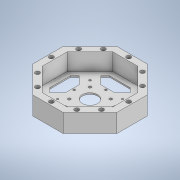
# Autodesk Inventor part: Base_Lid
Saved by Autodesk Inventor 2022 (Build 260153000, 153)
## iProperties
Created: 2022-03-24
Part Number: Base_Lid
Material: Generic
Document SubType Name: Modeling
Designer: Mlees
Density: 1 g/cm^3
Appearance: Default
Author: Mlees
Autodesk Inventor part; units mm, degrees
ref_plane "YZ Plane" through (0, 0, 0) normal (1, 0, 0) x (0, 1, 0)
ref_plane "XZ Plane" through (0, 0, 0) normal (0, 1, 0) x (-1, 0, 0)
ref_plane "XY Plane" through (0, 0, 0) normal (0, 0, 1) x (1, 0, 0)
sketch "Sketch1" plane through (0, 0, 0) normal (0, 1, 0) x (-1, 0, 0)
  line L0 (0, 0) -> (0, 22.75)
  line L1 (40, 62.75) -> (0, 22.75)
  line L2 (40, 62.75) -> (85.5, 62.75)
  line L3 (85.5, 62.75) -> (125.5, 22.75)
  line L4 (125.5, 22.75) -> (125.5, 0)
  line L5 (0, 0) -> (0, -22.75)
  line L6 (40, -62.75) -> (0, -22.75)
  line L7 (40, -62.75) -> (85.5, -62.75)
  line L8 (85.5, -62.75) -> (125.5, -22.75)
  line L9 (125.5, -22.75) -> (125.5, 0)
  dimension "d0" = 22.75
  dimension "d3" = 45.5
  dimension "d4" = 135
  constraints: 20 end point, 1 horizontal, 1 perpendicular, 1 vertical
  measures "d0" distance of L0.start L0.end
  measures "d3" distance of L1.start L2.end
  measures "d4" angle of L2 L3
extrude "Extrusion1" add sketch "Sketch1" along normal blind 2
sketch "Sketch2" plane through (0, 2, 0) normal (0, 1, 0) x (1, 0, 0)
  line L0 (-85.5, -62.75) -> (-40, -62.75) projected
  line L1 (-62.75, -62.75) -> (-62.75, 0)
  circle A0 centre (-62.75, 0) radius 11.5
  point P0 (0, 0)
  point P1 (-78.25, -15.5)
  point P2 (-47.25, -15.5)
  point P3 (-47.25, 15.5)
  point P4 (-78.25, 15.5)
  dimension "d7" = 23
  constraints: 2 end point, 1 centre point, 1 coincident, 1 midpoint, 1 vertical
  measures "d7" diameter of A0
extrude "Extrusion2" cut sketch "Sketch2" against normal blind 2
sketch "Sketch3" plane through (0, 2, 0) normal (0, 1, 0) x (1, 0, 0)
  circle A0 centre (-62.75, 0) radius 11.5 projected
  point P0 (0, 0)
  point P1 (-78.25, -15.5)
  point P2 (-47.25, -15.5)
  point P3 (-47.25, 15.5)
  point P4 (-78.25, 15.5)
hole "Hole1" at (-78.25, 2, 15.5) at (-47.25, 2, 15.5) at (-47.25, 2, -15.5) at (-78.25, 2, -15.5) direction (0, -1, 0) diameter 4 depth 2 tip angle 118
sketch "Sketch4" plane through (0, 2, 0) normal (0, 1, 0) x (1, 0, 0)
  line L0 (-125.5, -22.75) -> (-85.5, -62.75) projected
  line L1 (-85.5, -62.75) -> (-125.5, -22.75)
  line L2 (-125.5, 22.75) -> (-125.5, -22.75) projected
  line L3 (-125.5, -22.75) -> (-125.5, 22.75)
  line L4 (-85.5, 62.75) -> (-125.5, 22.75) projected
  line L5 (-125.5, 22.75) -> (-85.5, 62.75)
  line L6 (-40, 62.75) -> (-85.5, 62.75) projected
  line L7 (-85.5, 62.75) -> (-40, 62.75)
  line L8 (0, -22.75) -> (0, 22.75) projected
  line L9 (-40, 62.75) -> (0, 22.75)
  line L10 (0, 22.75) -> (0, -22.75)
  line L11 (-40, -62.75) -> (0, -22.75) projected
  line L12 (0, -22.75) -> (-40, -62.75)
  line L13 (-85.5, -62.75) -> (-40, -62.75) projected
  line L14 (-40, -62.75) -> (-85.5, -62.75)
  circle A0 centre (-62.75, 0) radius 11.5 projected
  point P0 (0, 0)
  point P1 (-62.75, -57.75)
  point P2 (-92.0542, -49.1247)
  point P3 (-110.5001, -30.6788)
  point P4 (-33.4458, -49.1247)
  point P5 (-14.9999, -30.6788)
  point P6 (-5, 0)
  point P7 (-120.5, 0)
  point P8 (-62.75, 57.75)
  point P9 (-92.0542, 49.1247)
  point P10 (-110.5001, 30.6788)
  point P11 (-33.4458, 49.1247)
  point P12 (-14.9999, 30.6788)
  constraints: 16 end point, 8 equal length
hole "Hole2" at (-62.75, 2, 57.75) at (-92.0542, 2, 49.1247) at (-110.5001, 2, 30.6788) at (-33.4458, 2, 49.1247) at (-14.9999, 2, 30.6788) at (-5, 2, 0) at (-120.5, 2, 0) at (-110.5001, 2, -30.6788) at (-92.0542, 2, -49.1247) at (-62.75, 2, -57.75) at (-33.4458, 2, -49.1247) at (-14.9999, 2, -30.6788) direction (0, -1, 0) diameter 4 depth 2 tip angle 118
sketch "Sketch5" plane through (0, 2, 0) normal (0, 1, 0) x (1, 0, 0)
  line L0 (-40, -62.75) -> (0, -22.75) projected
  line L1 (-85.5, -62.75) -> (-40, -62.75) projected
  line L2 (-40, -62.75) -> (-85.5, -62.75)
  line L3 (-125.5, 22.75) -> (-125.5, -22.75) projected
  line L4 (-85.5, -62.75) -> (-125.5, -22.75)
  line L5 (-125.5, -22.75) -> (-125.5, 22.75)
  line L6 (-85.5, 62.75) -> (-125.5, 22.75) projected
  line L7 (-125.5, 22.75) -> (-85.5, 62.75)
  line L8 (-40, 62.75) -> (-85.5, 62.75) projected
  line L9 (-85.5, 62.75) -> (-40, 62.75)
  line L10 (0, -22.75) -> (0, 22.75) projected
  line L11 (-40, 62.75) -> (0, 22.75)
  line L12 (0, 22.75) -> (0, -22.75)
  line L13 (0, -22.75) -> (-40, -62.75)
  line L14 (-81.3579, -52.75) -> (-44.1421, -52.75)
  line L15 (-10, -18.6079) -> (-10, 18.6079)
  line L16 (-44.1421, 52.75) -> (-81.3579, 52.75)
  line L17 (-115.5, 18.6079) -> (-115.5, -18.6079)
  line L18 (-49.1421, -18.6079) -> (-76.3579, -18.6079)
  line L19 (-81.3579, -13.6079) -> (-81.3579, 13.6079)
  line L20 (-76.3579, 18.6079) -> (-49.1421, 18.6079)
  line L21 (-44.1421, 13.6079) -> (-44.1421, -13.6079)
  line L22 (-44.1421, -13.6079) -> (-24.5711, -33.1789)
  line L23 (-49.1421, -18.6079) -> (-29.5711, -38.1789)
  line L24 (-76.3579, -18.6079) -> (-95.9289, -38.1789)
  line L25 (-81.3579, -13.6079) -> (-100.9289, -33.1789)
  line L26 (-81.3579, 13.6079) -> (-100.9289, 33.1789)
  line L27 (-76.3579, 18.6079) -> (-95.9289, 38.1789)
  line L28 (-49.1421, 18.6079) -> (-29.5711, 38.1789)
  line L29 (-44.1421, 13.6079) -> (-24.5711, 33.1789)
  line L30 (-115.5, -18.6079) -> (-100.9289, -33.1789)
  line L31 (-95.9289, -38.1789) -> (-81.3579, -52.75)
  line L32 (-44.1421, -52.75) -> (-29.5711, -38.1789)
  line L33 (-24.5711, -33.1789) -> (-10, -18.6079)
  line L34 (-10, 18.6079) -> (-24.5711, 33.1789)
  line L35 (-29.5711, 38.1789) -> (-44.1421, 52.75)
  line L36 (-91.6863, -38.1789) -> (-75.1152, -21.6079)
  line L37 (-75.1152, -21.6079) -> (-50.3848, -21.6079)
  line L38 (-50.3848, -21.6079) -> (-33.8137, -38.1789)
  line L39 (-33.8137, -38.1789) -> (-45.3848, -49.75)
  line L40 (-45.3848, -49.75) -> (-80.1152, -49.75)
  line L41 (-80.1152, -49.75) -> (-91.6863, -38.1789)
  line L42 (-81.3579, 52.75) -> (-95.9289, 38.1789)
  line L43 (-100.9289, 33.1789) -> (-115.5, 18.6079)
  line L44 (-100.9289, -28.9363) -> (-84.3579, -12.3652)
  line L45 (-84.3579, -12.3652) -> (-84.3579, 12.3652)
  line L46 (-84.3579, 12.3652) -> (-100.9289, 28.9363)
  line L47 (-100.9289, 28.9363) -> (-112.5, 17.3652)
  line L48 (-112.5, 17.3652) -> (-112.5, -17.3652)
  line L49 (-112.5, -17.3652) -> (-100.9289, -28.9363)
  line L50 (-91.6863, 38.1789) -> (-75.1152, 21.6079)
  line L51 (-75.1152, 21.6079) -> (-50.3848, 21.6079)
  line L52 (-50.3848, 21.6079) -> (-33.8137, 38.1789)
  line L53 (-33.8137, 38.1789) -> (-45.3848, 49.75)
  line L54 (-45.3848, 49.75) -> (-80.1152, 49.75)
  line L55 (-80.1152, 49.75) -> (-91.6863, 38.1789)
  line L56 (-41.1421, -12.3652) -> (-41.1421, 12.3652)
  line L57 (-41.1421, 12.3652) -> (-24.5711, 28.9363)
  line L58 (-24.5711, 28.9363) -> (-13, 17.3652)
  line L59 (-13, 17.3652) -> (-13, -17.3652)
  line L60 (-13, -17.3652) -> (-24.5711, -28.9363)
  line L61 (-24.5711, -28.9363) -> (-41.1421, -12.3652)
  line L62 (-73.0442, -26.6079) -> (-84.6152, -38.1789)
  line L63 (-84.6152, -38.1789) -> (-78.0442, -44.75)
  line L64 (-78.0442, -44.75) -> (-47.4558, -44.75)
  line L65 (-47.4558, -44.75) -> (-40.8848, -38.1789)
  line L66 (-40.8848, -38.1789) -> (-52.4558, -26.6079)
  line L67 (-52.4558, -26.6079) -> (-73.0442, -26.6079)
  line L68 (-100.9289, -21.8652) -> (-89.3579, -10.2942)
  line L69 (-89.3579, -10.2942) -> (-89.3579, 10.2942)
  line L70 (-89.3579, 10.2942) -> (-100.9289, 21.8652)
  line L71 (-100.9289, 21.8652) -> (-107.5, 15.2942)
  line L72 (-107.5, 15.2942) -> (-107.5, -15.2942)
  line L73 (-107.5, -15.2942) -> (-100.9289, -21.8652)
  line L74 (-73.0442, 26.6079) -> (-84.6152, 38.1789)
  line L75 (-84.6152, 38.1789) -> (-78.0442, 44.75)
  line L76 (-78.0442, 44.75) -> (-47.4558, 44.75)
  line L77 (-47.4558, 44.75) -> (-40.8848, 38.1789)
  line L78 (-40.8848, 38.1789) -> (-52.4558, 26.6079)
  line L79 (-52.4558, 26.6079) -> (-73.0442, 26.6079)
  line L80 (-36.1421, 10.2942) -> (-36.1421, -10.2942)
  line L81 (-36.1421, -10.2942) -> (-24.5711, -21.8652)
  line L82 (-24.5711, -21.8652) -> (-18, -15.2942)
  line L83 (-18, -15.2942) -> (-18, 15.2942)
  line L84 (-18, 15.2942) -> (-24.5711, 21.8652)
  line L85 (-24.5711, 21.8652) -> (-36.1421, 10.2942)
  point P0 (0, 0)
  dimension "d39" = 3
  dimension "d40" = 3
  dimension "d41" = 3
  dimension "d42" = 3
  dimension "d59" = 7.0711
  dimension "d60" = 7.0711
  dimension "d61" = 5
  dimension "d62" = 5
  dimension "d63" = 5
  dimension "d64" = 5
  constraints: 160 end point, 33 perpendicular, 8 point on line, 6 equal length, 1 horizontal, 40 other
  measures "d39" distance between parallel lines of L24 L36
  measures "d40" distance between parallel lines of L30 L49
  measures "d41" distance between parallel lines of L27 L50
  measures "d42" distance between parallel lines of L21 L56
  measures "d59" distance between parallel lines of L25 L24
  measures "d60" distance between parallel lines of L27 L26
  measures "d61" distance between parallel lines of L36 L62
  measures "d62" distance between parallel lines of L49 L73
  measures "d63" distance between parallel lines of L50 L74
  measures "d64" distance between parallel lines of L56 L80
extrude "Extrusion3" cut sketch "Sketch5" against normal blind 2 contours L67 L66 L65 L64 L63 L62 | L73 L72 L71 L70 L69 L68 | L74 L75 L76 L77 L78 L79 | L85 L84 L83 L82 L81 L80
sketch "Sketch6" plane through (0, 2, 0) normal (0, 1, 0) x (1, 0, 0)
  line L0 (-85.5, -62.75) -> (-40, -62.75) projected
  line L1 (-125.5, -22.75) -> (-85.5, -62.75) projected
  line L2 (-40, -62.75) -> (-85.5, -62.75)
  line L3 (-85.5, -62.75) -> (-125.5, -22.75)
  line L4 (-85.5, 62.75) -> (-125.5, 22.75) projected
  line L5 (-125.5, -22.75) -> (-125.5, 22.75)
  line L6 (-125.5, 22.75) -> (-85.5, 62.75)
  line L7 (-40, 62.75) -> (-85.5, 62.75) projected
  line L8 (-85.5, 62.75) -> (-40, 62.75)
  line L9 (0, -22.75) -> (0, 22.75) projected
  line L10 (-40, 62.75) -> (0, 22.75)
  line L11 (0, 22.75) -> (0, -22.75)
  line L12 (-40, -62.75) -> (0, -22.75) projected
  line L13 (0, -22.75) -> (-40, -62.75)
  line L14 (-115.5, 18.6079) -> (-115.5, -18.6079)
  line L15 (-115.5, -18.6079) -> (-81.3579, -52.75)
  line L16 (-81.3579, -52.75) -> (-44.1421, -52.75)
  line L17 (-44.1421, -52.75) -> (-10, -18.6079)
  line L18 (-10, -18.6079) -> (-10, 18.6079)
  line L19 (-10, 18.6079) -> (-44.1421, 52.75)
  line L20 (-44.1421, 52.75) -> (-81.3579, 52.75)
  line L21 (-81.3579, 52.75) -> (-115.5, 18.6079)
  circle A0 centre (-62.75, -57.75) radius 2 projected
  circle A1 centre (-62.75, -57.75) radius 3.25
  circle A2 centre (-92.0542, -49.1247) radius 2 projected
  circle A3 centre (-92.0542, -49.1247) radius 3.25
  circle A4 centre (-110.5001, -30.6788) radius 2 projected
  circle A5 centre (-110.5001, -30.6788) radius 3.25
  circle A6 centre (-120.5, 0) radius 2 projected
  circle A7 centre (-120.5, 0) radius 3.25
  circle A8 centre (-110.5001, 30.6788) radius 2 projected
  circle A9 centre (-110.5001, 30.6788) radius 3.25
  circle A10 centre (-92.0542, 49.1247) radius 2 projected
  circle A11 centre (-92.0542, 49.1247) radius 3.25
  circle A12 centre (-62.75, 57.75) radius 2 projected
  circle A13 centre (-62.75, 57.75) radius 3.25
  circle A14 centre (-33.4458, 49.1247) radius 2 projected
  circle A15 centre (-33.4458, 49.1247) radius 3.25
  circle A16 centre (-14.9999, 30.6788) radius 2 projected
  circle A17 centre (-14.9999, 30.6788) radius 3.25
  circle A18 centre (-5, 0) radius 2 projected
  circle A19 centre (-5, 0) radius 3.25
  circle A20 centre (-14.9999, -30.6788) radius 2 projected
  circle A21 centre (-14.9999, -30.6788) radius 3.25
  circle A22 centre (-33.4458, -49.1247) radius 2 projected
  circle A23 centre (-33.4458, -49.1247) radius 3.25
  point P0 (0, 0)
  dimension "d45" = 10
  dimension "d46" = 6.5
  dimension "d47" = 6.5
  dimension "d48" = 6.5
  dimension "d49" = 6.5
  constraints: 32 end point, 12 centre point, 12 coincident, 6 equal length, 4 perpendicular, 1 horizontal, 7 other
  measures "d45" distance between parallel lines of L5 L14
  measures "d46" diameter of A1
  measures "d47" diameter of A3
  measures "d48" diameter of A5
  measures "d49" diameter of A7
extrude "Extrusion4" add sketch "Sketch6" along normal blind 25.4 contours L1 L5 L4 L7 L10 L9 L12 L0
sketch "Sketch8" plane through (0, 0, 0) normal (0, -1, 0) x (1, 0, 0)
  line L0 (-52.4558, 26.6079) -> (-73.0442, 26.6079) projected
  circle A0 centre (-62.75, 0) radius 11.5 projected
  circle A1 centre (-62.75, 0) radius 11.5
  line L1 (-73.0442, 26.6079) -> (-84.6152, 38.1789) projected
  line L2 (-100.9289, 21.8652) -> (-89.3579, 10.2942) projected
  line L3 (-36.1421, -10.2942) -> (-36.1421, 10.2942) projected
  line L4 (-73.0442, -26.6079) -> (-52.4558, -26.6079) projected
  line L5 (-89.3579, 10.2942) -> (-89.3579, -10.2942) projected
  point P0 (0, 0)
  point P1 (-39.1421, 0)
  point P2 (-62.75, -23.6079)
  point P3 (-86.3579, 0)
  point P4 (-62.75, 23.6079)
  point P5 (-86.9865, 24.2366)
  point P6 (-38.5134, 24.2365)
  point P7 (-38.5135, -24.2366)
  point P8 (-86.9866, -24.2365)
  dimension "d82" = 3
  dimension "d83" = 3
  dimension "d84" = 3
  dimension "d85" = 3
  constraints: 1 centre point, 1 coincident
  measures "d82" distance from line of point (-62.75, 23.608) L0
  measures "d83" distance from line of point (-39.142, 0) L3
  measures "d84" distance from line of L4 point (-62.75, -23.608)
  measures "d85" distance from line of L5 point (-86.358, 0)
hole "Hole4" at (-39.1421, 0, 0) at (-62.75, 0, -23.6079) at (-86.3579, 0, 0) at (-62.75, 0, 23.6079) at (-86.9865, 0, 24.2366) at (-38.5134, 0, 24.2365) at (-38.5135, 0, -24.2366) at (-86.9866, 0, -24.2365) direction (0, 1, 0) diameter 3 depth 2 tip angle 118
body "Solid1"
